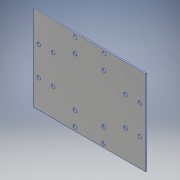
# Autodesk Inventor part: base_diff_02
Saved by Autodesk Inventor 2018.1 (Build 221171000, 171)
## iProperties
Created: 2017-09-21
Part Number: base_diff_02
Material: アルミニウム 6061
Document SubType Name: Modeling
Designer: Kakeru Yamashita
Density: 2.7 g/cm^3
Appearance: アルミニウム - フラット
Author: Kakeru Yamashita
Autodesk Inventor part; units mm, degrees
ref_plane "YZ Plane" through (0, 0, 0) normal (1, 0, 0) x (0, 1, 0)
ref_plane "XZ Plane" through (0, 0, 0) normal (0, 1, 0) x (-1, 0, 0)
ref_plane "XY Plane" through (0, 0, 0) normal (0, 0, 1) x (1, 0, 0)
sketch "スケッチ1" plane through (0, 0, 0) normal (0, 1, 0) x (-1, 0, 0)
  line L0 (0, 0) -> (310, 0)
  line L1 (310, 0) -> (310, -235)
  line L2 (310, -235) -> (0, -235)
  line L3 (0, -235) -> (0, 0)
  dimension "d0" = 310
  dimension "d1" = 235
  constraints: 8 end point, 2 parallel, 1 horizontal, 1 perpendicular
  measures "d0" distance of L1.end L2.end
  measures "d1" distance of L2.end L0.start
extrude "押し出し1" add sketch "スケッチ1" along normal blind 3
sketch "スケッチ2" plane through (0, 3, 0) normal (0, 1, 0) x (1, 0, 0)
  line L0 (-155, -40) -> (-155, 284.5269)
  line L1 (-155, 284.5269) -> (-194.2717, 284.5269)
  line L2 (30, 117.5) -> (-350, 117.5)
  line L3 (0, 0) -> (0, 235) projected
  line L4 (-310, 0) -> (0, 0) projected
  circle A0 centre (-195, 10) radius 5
  circle A1 centre (-115, 10) radius 5
  circle A2 centre (-195, 225) radius 5
  circle A3 centre (-115, 225) radius 5
  circle A4 centre (-195, 50) radius 5
  circle A5 centre (-115, 50) radius 5
  circle A6 centre (-195, 185) radius 5
  circle A7 centre (-115, 185) radius 5
  circle A8 centre (-295, 157.5) radius 5
  line L5 (-310, 235) -> (-310, 0) projected
  circle A9 centre (-295, 77.5) radius 5
  circle A10 centre (-15, 157.5) radius 5
  circle A11 centre (-15, 77.5) radius 5
  circle A12 centre (-255, 157.5) radius 5
  circle A13 centre (-255, 77.5) radius 5
  circle A14 centre (-55, 157.5) radius 5
  circle A15 centre (-55, 77.5) radius 5
  dimension "d4" = 155
  dimension "d5" = 117.5
  dimension "d6" = 10
  dimension "d7" = 40
  dimension "d8" = 10
  dimension "d9" = 10
  dimension "d10" = 40
  dimension "d11" = 10
  dimension "d12" = 15
  dimension "d13" = 40
  dimension "d14" = 10
  dimension "d15" = 40
  constraints: 16 centre point, 12 symmetric about line, 6 end point, 1 horizontal, 1 horizontal alignment, 1 perpendicular, 1 vertical, 1 vertical alignment, 12 other
  measures "d4" distance between parallel lines of L3 L0
  measures "d5" distance between parallel lines of L4 L2
  measures "d6" diameter of A0
  measures "d7" distance from line of L0 A0.centre
  measures "d8" distance from line of L4 A0.centre
  measures "d9" diameter of A4
  measures "d10" distance of A4.centre A0.centre
  measures "d11" diameter of A8
  measures "d12" distance from line of L5 A8.centre
  measures "d13" distance from line of L2 A8.centre
  measures "d14" diameter of A12
  measures "d15" distance of A12.centre A8.centre
extrude "押し出し2" cut sketch "スケッチ2" against normal blind 3 contours A0 | A1 | A2 | A3 | A4 | A5 | A6 | A7 | A8 | A9 | A10 | A11 | A12 | A13 | A14 | A15
